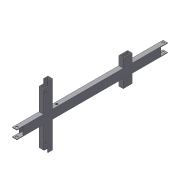
# Autodesk Inventor part: Frame_MainStructuralMember
Saved by Autodesk Inventor 2012 (Build 160160000, 160)
## iProperties
Created: 2012-01-13
Part Number: Frame_MainStructuralMember
Material: Aluminum-6061
Document SubType Name: Modeling
Designer: JesseK
Mass: 1397.7 g
Surface Area: 3299.42 cm^2
Volume: 515.755 cm^3
Density: 2.71 g/cm^3
Author: JesseK
Autodesk Inventor part; units mm, degrees
ref_plane "YZ Plane" through (0, 0, 0) normal (1, 0, 0) x (0, 1, 0)
ref_plane "XZ Plane" through (0, 0, 0) normal (0, 1, 0) x (-1, 0, 0)
ref_plane "XY Plane" through (0, 0, 0) normal (0, 0, 1) x (1, 0, 0)
sketch "Sketch1" plane through (0, 0, 0) normal (0, 0, 1) x (1, 0, 0)
  line L0 (0, 0) -> (25.4, 0)
  line L1 (25.4, 0) -> (25.4, 50.8)
  line L2 (25.4, 50.8) -> (0, 50.8)
  line L3 (0, 50.8) -> (0, 0)
  dimension "d0" = 25.4
  dimension "d1" = 50.8
  constraints: 8 end point, 2 parallel, 1 horizontal, 1 perpendicular
  measures "d0" distance of L1.end L2.end
  measures "d1" distance of L0.end L1.end
extrude "Extrusion1" add sketch "Sketch1" along normal blind 863.6
sketch "Sketch2" plane through (0, 50.8, 0) normal (0, 1, 0) x (1, 0, 0)
  line L0 (0, -863.6) -> (25.4, -863.6) projected
  line L1 (25.4, 0) -> (25.4, -863.6) projected
  line L2 (0, 0) -> (0, -863.6) projected
  line L3 (0, -203.2) -> (25.4, -203.2)
  line L4 (25.4, -203.2) -> (25.4, -254)
  line L5 (25.4, -254) -> (0, -254)
  line L6 (0, -254) -> (0, -203.2)
  dimension "d5" = 50.8
  dimension "d6" = 609.6
  constraints: 8 end point, 2 parallel, 2 point on line, 1 horizontal, 1 perpendicular
  measures "d5" distance of L3.end L4.end
  measures "d6" distance between parallel lines of L0 L5
extrude "Extrusion2" add sketch "Sketch2" along normal blind 50.8 and the other way blind 101.6 contours L2 L3 L1 L5
sketch "Sketch4" plane through (0, 50.8, 863.6) normal (0, 1, 0) x (1, 0, 0)
  line L0 (0, 609.6) -> (0, 0) projected
  line L1 (0, 0) -> (25.4, 0) projected
  line L2 (25.4, 609.6) -> (25.4, 0) projected
  line L3 (0, 203.2) -> (25.4, 203.2)
  line L4 (25.4, 203.2) -> (25.4, 152.4)
  line L5 (25.4, 152.4) -> (0, 152.4)
  line L6 (0, 152.4) -> (0, 203.2)
  point P0 (0, 863.6)
  dimension "d14" = 50.8
  dimension "d15" = 152.4
  constraints: 8 end point, 2 parallel, 2 point on line, 1 horizontal, 1 perpendicular
  measures "d14" distance of L3.end L4.end
  measures "d15" distance between parallel lines of L1 L5
extrude "Extrusion4" add sketch "Sketch4" along normal blind 152.4 and the other way blind 203.2 contours L3 L2 L5 L0
shell "Shell3" thickness 3.175 removed faces 6 at (8.4667, 33.8667, 0) at (8.4667, -50.8, 220.1333) at (8.4667, 101.6, 220.1333) at (16.9333, -152.4, 694.2667) at (8.4667, 33.8667, 863.6) at (16.9333, 203.2, 694.2667)
sketch "Sketch5" plane through (25.4, 0, 0) normal (1, 0, 0) x (0, 0, -1)
  line L0 (-863.6, 50.8) -> (-863.6, 0) projected
  line L1 (0, 0) -> (-203.2, 0) projected
  line L2 (0, 0) -> (0, 50.8) projected
  line L3 (0, 47.625) -> (-38.1, 47.625)
  line L4 (-38.1, 47.625) -> (-38.1, 3.175)
  line L5 (-38.1, 3.175) -> (0, 3.175)
  line L6 (0, 3.175) -> (0, 47.625)
  line L7 (-863.6, 47.625) -> (-825.5, 47.625)
  line L8 (-825.5, 47.625) -> (-825.5, 3.175)
  line L9 (-825.5, 3.175) -> (-863.6, 3.175)
  line L10 (-863.6, 3.175) -> (-863.6, 47.625)
  dimension "d23" = 44.45
  dimension "d24" = 3.175
  dimension "d25" = 38.1
  constraints: 16 end point, 4 parallel, 3 collinear, 2 horizontal, 2 perpendicular, 2 point on line
  measures "d23" distance of L3.end L4.end
  measures "d24" distance between parallel lines of L1 L5
  measures "d25" distance of L4.end L5.end
extrude "Extrusion5" cut sketch "Sketch5" against normal through all
sketch "Sketch6" plane through (0, 0, 0) normal (0, -1, 0) x (1, 0, 0)
  line L0 (0, 0) -> (0, 203.2) projected
  line L1 (0, 0) -> (25.4, 0) projected
  circle A0 centre (12.7, 12.7) radius 6.35
  dimension "d28" = 12.7
  dimension "d29" = 12.7
  dimension "d30" = 12.7
  constraints: 1 centre point
  measures "d28" distance from line of L1 A0.centre
  measures "d29" distance from line of L0 A0.centre
  measures "d30" diameter of A0
extrude "Extrusion6" cut sketch "Sketch6" against normal through all
sketch "Sketch7" plane through (0, 0, 863.6) normal (0, -1, 0) x (1, 0, 0)
  line L0 (25.4, -152.4) -> (25.4, 0) projected
  line L1 (25.4, 0) -> (0, 0) projected
  circle A0 centre (12.7, -12.7) radius 6.35
  point P0 (0, -863.6)
  dimension "d33" = 12.7
  dimension "d34" = 12.7
  dimension "d35" = 12.7
  constraints: 1 centre point
  measures "d33" diameter of A0
  measures "d34" distance from line of L1 A0.centre
  measures "d35" distance from line of L0 A0.centre
extrude "Extrusion7" cut sketch "Sketch7" against normal through all
sketch "Sketch8" plane through (25.4, -50.8, 254) normal (1, 0, 0) x (0, 0, -1)
  line L0 (-457.2, 254) -> (-431.8, 254)
  line L1 (-431.8, 254) -> (-431.8, 228.6)
  line L2 (-431.8, 228.6) -> (-457.2, 228.6)
  line L3 (-457.2, 228.6) -> (-457.2, 254)
  line L4 (-457.2, -101.6) -> (-431.8, -101.6)
  line L5 (-431.8, -101.6) -> (-431.8, -76.2)
  line L6 (-431.8, -76.2) -> (-457.2, -76.2)
  line L7 (-457.2, -76.2) -> (-457.2, -101.6)
  dimension "d38" = 25.4
  dimension "d39" = 25.4
  constraints: 16 end point, 4 parallel, 2 collinear, 2 horizontal, 2 perpendicular
  measures "d38" distance of L4.end L5.end
  measures "d39" distance of L5.end L6.end
extrude "Extrusion8" cut sketch "Sketch8" against normal through all
sketch "Sketch9" plane through (25.4, -50.8, 254) normal (1, 0, 0) x (0, 0, -1)
  line L0 (-431.8, 228.6) -> (-457.2, 228.6) projected
  line L1 (-457.2, 101.6) -> (-457.2, 228.6) projected
  line L2 (-457.2, -76.2) -> (-457.2, 50.8) projected
  line L3 (-457.2, -76.2) -> (-431.8, -76.2) projected
  circle A0 centre (-444.5, 203.2) radius 6.35
  circle A1 centre (-444.5, -50.8) radius 6.35
  dimension "d42" = 12.7
  dimension "d43" = 25.4
  dimension "d44" = 12.7
  dimension "d45" = 25.4
  dimension "d46" = 12.7
  constraints: 2 centre point, 1 equal radius
  measures "d42" diameter of A0
  measures "d43" distance from line of L0 A0.centre
  measures "d44" distance from line of L1 A0.centre
  measures "d45" distance from line of L3 A1.centre
  measures "d46" distance from line of L2 A1.centre
extrude "Extrusion9" cut sketch "Sketch9" against normal through all
sketch "Sketch10" plane through (0, 50.8, 254) normal (0, 1, 0) x (1, 0, 0)
  line L0 (0, -406.4) -> (25.4, -406.4) projected
  line L1 (25.4, 0) -> (25.4, -406.4) projected
  circle A0 centre (12.7, -368.3) radius 6.35
  point P0 (0, 254)
  dimension "d49" = 12.7
  dimension "d50" = 12.7
  dimension "d51" = 38.1
  constraints: 1 centre point
  measures "d49" diameter of A0
  measures "d50" distance from line of L1 A0.centre
  measures "d51" distance from line of L0 A0.centre
extrude "Extrusion10" cut sketch "Sketch10" against normal through all
body "Solid1"
